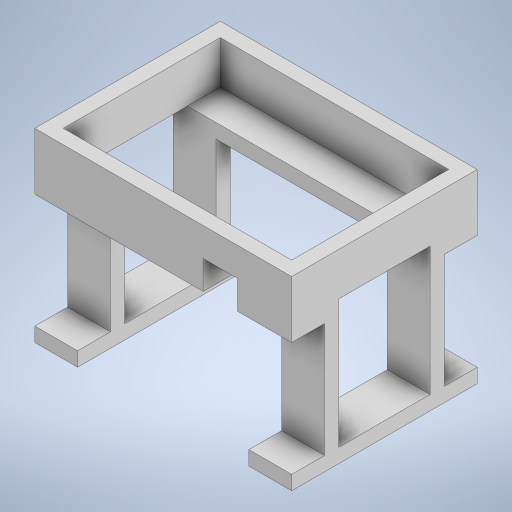
# Autodesk Inventor part: gcs microhard
Saved by Autodesk Inventor 2023 (Build 270158000, 158)
## iProperties
Created: 2022-10-22
Part Number: gcs microhard
Material: Generic
Document SubType Name: Modeling
Designer: Eli
Density: 1 g/cm^3
Appearance: Default
Author: Eli
Autodesk Inventor part; units mm, degrees
ref_plane "YZ Plane" through (0, 0, 0) normal (1, 0, 0) x (0, 1, 0)
ref_plane "XZ Plane" through (0, 0, 0) normal (0, 1, 0) x (-1, 0, 0)
ref_plane "XY Plane" through (0, 0, 0) normal (0, 0, 1) x (1, 0, 0)
sketch "Sketch1" plane through (0, 0, 0) normal (0, 1, 0) x (-1, 0, 0)
  line L0 (0, 0) -> (-57.15, 0)
  line L1 (-57.15, 0) -> (-57.15, -41.275)
  line L2 (-57.15, -41.275) -> (0, -41.275)
  line L3 (0, -41.275) -> (0, 0)
  line L4 (-3.175, -3.175) -> (-53.975, -3.175)
  line L5 (-53.975, -3.175) -> (-53.975, -38.1)
  line L6 (-53.975, -38.1) -> (-3.175, -38.1)
  line L7 (-3.175, -38.1) -> (-3.175, -3.175)
  line L8 (0, -20.6375) -> (-57.15, -20.6375) construction
  line L9 (-28.575, 0) -> (-28.575, -41.275) construction
  point P0 (-3.175, -20.6375)
  dimension "d0" = 57.15
  dimension "d1" = 41.275
  dimension "d2" = 3.175
  dimension "d3" = 3.175
  constraints: 20 end point, 5 midpoint, 4 parallel, 2 horizontal, 2 perpendicular, 2 other
  measures "d0" distance of L1.end L2.end
  measures "d1" distance of L0.end L1.end
  measures "d2" distance between parallel lines of L0 L4
  measures "d3" distance from line of L3 point (-3.175, -20.637)
extrude "Extrusion4" add sketch "Sketch1" along normal blind 9.525
sketch "Sketch4" plane through (57.15, 0, 0) normal (1, 0, 0) x (0, 0, -1)
  line L0 (0, 0) -> (0, 9.525) projected
  line L1 (0, 0) -> (10.4775, 0)
  line L2 (10.4775, 0) -> (10.4775, -3.175)
  line L3 (10.4775, -3.175) -> (0, -3.175)
  line L4 (0, -3.175) -> (0, 0)
  line L5 (41.275, 0) -> (41.275, 9.525) projected
  line L6 (41.275, 0) -> (30.7975, 0)
  line L7 (30.7975, 0) -> (30.7975, -3.175)
  line L8 (30.7975, -3.175) -> (41.275, -3.175)
  line L9 (41.275, -3.175) -> (41.275, 0)
  line L10 (3.175, 9.525) -> (38.1, 9.525) construction
  line L11 (20.6375, 9.525) -> (20.6375, 0) construction
  line L12 (3.175, 0) -> (38.1, 0) construction
  dimension "d25" = 20.32
  dimension "d26" = 3.175
  constraints: 18 end point, 4 parallel, 2 horizontal, 2 midpoint, 2 perpendicular, 1 point on line, 1 other
  measures "d25" distance between parallel lines of L7 L2
  measures "d26" distance between parallel lines of L1 L3
extrude "Extrusion5" add sketch "Sketch4" against normal up to surface (57.15 mm away)
sketch "Sketch5" plane through (0, 9.525, 0) normal (0, 0, 1) x (1, 0, 0)
  line L0 (57.15, -12.7) -> (0, -12.7) projected
  line L1 (37.465, -12.7) -> (45.085, -12.7)
  line L2 (45.085, -12.7) -> (45.085, -6.35)
  line L3 (45.085, -6.35) -> (37.465, -6.35)
  line L4 (37.465, -6.35) -> (37.465, -12.7)
  line L5 (53.975, -9.525) -> (53.975, 0) projected
  line L6 (0, -12.7) -> (0, 0) projected
  line L7 (3.175, -9.525) -> (3.175, 0) projected
  point P0 (0, -9.525)
  dimension "d29" = 16.51
  dimension "d31" = 41.91
  dimension "d32" = 6.35
  constraints: 8 end point, 2 parallel, 1 horizontal, 1 perpendicular, 1 point on line
  measures "d29" distance between parallel lines of L5 L4
  measures "d31" distance between parallel lines of L2 L7
  measures "d32" distance of L1.end L2.end
extrude "Extrusion6" cut sketch "Sketch5" against normal up to surface (10.4775 mm away)
sketch "Sketch6" plane through (57.15, -3.175, -41.275) normal (0, -1, 0) x (1, 0, 0)
  point P0 (-57.15, 41.275)
sketch "Sketch7" plane through (57.15, -3.175, -41.275) normal (0, -1, 0) x (1, 0, 0)
  line L0 (-3.175, 10.4775) -> (0, 10.4775) projected
  line L1 (0, 10.4775) -> (-9.525, 10.4775)
  line L2 (-9.525, 10.4775) -> (-9.525, 7.3025)
  line L3 (-9.525, 7.3025) -> (0, 7.3025)
  line L4 (0, 7.3025) -> (0, 10.4775)
  line L5 (0, 41.275) -> (0, 0) construction
  line L6 (0, 20.6375) -> (-57.15, 20.6375) construction
  line L7 (-57.15, 0) -> (-57.15, 41.275) construction
  line L8 (0, 30.7975) -> (-9.525, 30.7975)
  line L9 (-9.525, 30.7975) -> (-9.525, 33.9725)
  line L10 (-9.525, 33.9725) -> (0, 33.9725)
  line L11 (0, 33.9725) -> (0, 30.7975)
  line L12 (0, 0) -> (-57.15, 0) construction
  line L13 (-28.575, 0) -> (-28.575, 41.275) construction
  line L14 (-19.685, 41.275) -> (-57.15, 41.275) construction
  line L15 (-57.15, 10.4775) -> (-47.625, 10.4775)
  line L16 (-47.625, 10.4775) -> (-47.625, 7.3025)
  line L17 (-47.625, 7.3025) -> (-57.15, 7.3025)
  line L18 (-57.15, 7.3025) -> (-57.15, 10.4775)
  line L19 (-57.15, 41.275) -> (-57.15, 0) construction
  line L20 (-57.15, 30.7975) -> (-47.625, 30.7975)
  line L21 (-47.625, 30.7975) -> (-47.625, 33.9725)
  line L22 (-47.625, 33.9725) -> (-57.15, 33.9725)
  line L23 (-57.15, 33.9725) -> (-57.15, 30.7975)
  dimension "d35" = 3.175
  dimension "d36" = 9.525
  constraints: 38 end point, 12 symmetric about line, 3 midpoint, 2 parallel, 1 horizontal, 1 perpendicular, 1 point on line, 1 vertical
  measures "d35" distance of L3.end L0.end
  measures "d36" distance of L2.end L3.end
extrude "Extrusion7" add sketch "Sketch7" along normal blind 28.575
sketch "Sketch8" plane through (0, -3.175, -7.3025) normal (0, 0, 1) x (1, 0, 0)
  point P0 (0, 3.175)
sketch "Sketch9" plane through (0, 9.525, 0) normal (0, 0, 1) x (1, 0, 0)
  line L0 (0, -12.7) -> (0, -41.275) projected
  line L1 (9.525, -12.7) -> (9.525, -41.275) projected
  line L2 (0, -41.275) -> (9.525, -41.275)
  line L3 (9.525, -41.275) -> (9.525, -38.1)
  line L4 (9.525, -38.1) -> (0, -38.1)
  line L5 (0, -38.1) -> (0, -41.275)
  line L6 (57.15, -41.275) -> (57.15, -9.525) projected
  line L7 (47.625, -12.7) -> (47.625, -41.275) projected
  line L8 (57.15, -41.275) -> (47.625, -41.275)
  line L9 (47.625, -41.275) -> (47.625, -38.1)
  line L10 (47.625, -38.1) -> (57.15, -38.1)
  line L11 (57.15, -38.1) -> (57.15, -41.275)
  point P0 (0, -9.525)
  point P1 (0, -38.1)
  dimension "d39" = 3.175
  constraints: 16 end point, 4 parallel, 2 horizontal, 2 perpendicular, 2 point on line, 1 collinear
  measures "d39" distance between parallel lines of L2 L4
extrude "Extrusion8" add sketch "Sketch9" against normal up to surface (41.275 mm away)
body "Solid2"
